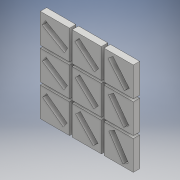
# Autodesk Inventor part: magnet-54-offset-9
Saved by Autodesk Inventor 2018 (Build 220112000, 112)
## iProperties
Created: 2025-03-17
Part Number: magnet-54-offset-9
Material: Generic
Document SubType Name: Modeling
Designer: neo
Density: 1 g/cm^3
Appearance: Default
Author: neo
Autodesk Inventor part; units mm, degrees
ref_plane "YZ Plane" through (0, 0, 0) normal (1, 0, 0) x (0, 1, 0)
ref_plane "XZ Plane" through (0, 0, 0) normal (0, 1, 0) x (-1, 0, 0)
ref_plane "XY Plane" through (0, 0, 0) normal (0, 0, 1) x (1, 0, 0)
sketch "Sketch1" plane through (0, 0, 0) normal (0, 1, 0) x (-1, 0, 0)
  line L0 (44.286, 57.5056) -> (-1.714, 57.5056)
  line L1 (-1.714, 57.5056) -> (-1.714, 11.5056)
  line L2 (-1.714, 11.5056) -> (44.286, 11.5056)
  line L3 (44.286, 11.5056) -> (44.286, 57.5056)
  line L4 (21.286, 57.5056) -> (21.286, 11.5056) construction
  line L5 (44.286, 34.5056) -> (-1.714, 34.5056) construction
  line L6 (32.0821, 50.9202) -> (21.286, 34.5056) construction
  line L7 (21.286, 34.5056) -> (12.8023, 40.0854) construction
  line L8 (36.6614, 48.5107) -> (28.0558, 54.1706)
  line L9 (28.0558, 54.1706) -> (5.9106, 20.5005)
  line L10 (5.9106, 20.5005) -> (14.5162, 14.8405)
  line L11 (14.5162, 14.8405) -> (36.6614, 48.5107)
  line L12 (94.286, 57.5056) -> (48.286, 57.5056)
  line L13 (48.286, 57.5056) -> (48.286, 11.5056)
  line L14 (48.286, 11.5056) -> (94.286, 11.5056)
  line L15 (94.286, 11.5056) -> (94.286, 57.5056)
  line L16 (71.286, 57.5056) -> (71.286, 11.5056) construction
  line L17 (94.286, 34.5056) -> (48.286, 34.5056) construction
  line L18 (84.7685, 48.7961) -> (71.286, 34.5056) construction
  line L19 (71.286, 34.5056) -> (63.9001, 41.4738) construction
  line L20 (88.8597, 45.628) -> (81.3678, 52.6963)
  line L21 (81.3678, 52.6963) -> (53.7123, 23.3831)
  line L22 (53.7123, 23.3831) -> (61.2042, 16.3148)
  line L23 (61.2042, 16.3148) -> (88.8597, 45.628)
  line L24 (144.286, 57.5056) -> (98.286, 57.5056)
  line L25 (98.286, 57.5056) -> (98.286, 11.5056)
  line L26 (98.286, 11.5056) -> (144.286, 11.5056)
  line L27 (144.286, 11.5056) -> (144.286, 57.5056)
  line L28 (121.286, 57.5056) -> (121.286, 11.5056) construction
  line L29 (144.286, 34.5056) -> (98.286, 34.5056) construction
  line L30 (137.0452, 46.2378) -> (121.286, 34.5056) construction
  line L31 (121.286, 34.5056) -> (115.2223, 42.6505) construction
  line L32 (140.5241, 42.4074) -> (134.3734, 50.6693)
  line L33 (134.3734, 50.6693) -> (102.0478, 26.6038)
  line L34 (102.0478, 26.6038) -> (108.1986, 18.3419)
  line L35 (108.1986, 18.3419) -> (140.5241, 42.4074)
  line L36 (44.286, 107.5056) -> (-1.714, 107.5056)
  line L37 (-1.714, 107.5056) -> (-1.714, 61.5056)
  line L38 (-1.714, 61.5056) -> (44.286, 61.5056)
  line L39 (44.286, 61.5056) -> (44.286, 107.5056)
  line L40 (21.286, 107.5056) -> (21.286, 61.5056) construction
  line L41 (44.286, 84.5056) -> (-1.714, 84.5056) construction
  line L42 (33.0183, 100.2647) -> (21.286, 84.5056) construction
  line L43 (21.286, 84.5056) -> (13.141, 90.5693) construction
  line L44 (37.4497, 97.593) -> (29.1878, 103.7437)
  line L45 (29.1878, 103.7437) -> (5.1223, 71.4182)
  line L46 (5.1223, 71.4182) -> (13.3842, 65.2674)
  line L47 (13.3842, 65.2674) -> (37.4497, 97.593)
  line L48 (44.286, 157.5056) -> (-1.714, 157.5056)
  line L49 (-1.714, 157.5056) -> (-1.714, 111.5056)
  line L50 (-1.714, 111.5056) -> (44.286, 111.5056)
  line L51 (44.286, 111.5056) -> (44.286, 157.5056)
  line L52 (21.286, 157.5056) -> (21.286, 111.5056) construction
  line L53 (44.286, 134.5056) -> (-1.714, 134.5056) construction
  line L54 (33.9147, 149.5559) -> (21.286, 134.5056) construction
  line L55 (21.286, 134.5056) -> (13.5074, 141.0326) construction
  line L56 (38.1833, 146.631) -> (30.293, 153.2517)
  line L57 (30.293, 153.2517) -> (4.3887, 122.3801)
  line L58 (4.3887, 122.3801) -> (12.279, 115.7594)
  line L59 (12.279, 115.7594) -> (38.1833, 146.631)
  line L60 (94.286, 107.5056) -> (48.286, 107.5056)
  line L61 (48.286, 107.5056) -> (48.286, 61.5056)
  line L62 (48.286, 61.5056) -> (94.286, 61.5056)
  line L63 (94.286, 61.5056) -> (94.286, 107.5056)
  line L64 (71.286, 107.5056) -> (71.286, 61.5056) construction
  line L65 (94.286, 84.5056) -> (48.286, 84.5056) construction
  line L66 (85.5766, 97.988) -> (71.286, 84.5056) construction
  line L67 (71.286, 84.5056) -> (64.3177, 91.8915) construction
  line L68 (89.4767, 94.5874) -> (82.4084, 102.0793)
  line L69 (82.4084, 102.0793) -> (53.0953, 74.4238)
  line L70 (53.0953, 74.4238) -> (60.1636, 66.9318)
  line L71 (60.1636, 66.9318) -> (89.4767, 94.5874)
  line L72 (94.286, 157.5056) -> (48.286, 157.5056)
  line L73 (48.286, 157.5056) -> (48.286, 111.5056)
  line L74 (48.286, 111.5056) -> (94.286, 111.5056)
  line L75 (94.286, 111.5056) -> (94.286, 157.5056)
  line L76 (71.286, 157.5056) -> (71.286, 111.5056) construction
  line L77 (94.286, 134.5056) -> (48.286, 134.5056) construction
  line L78 (86.3363, 147.1343) -> (71.286, 134.5056) construction
  line L79 (71.286, 134.5056) -> (64.759, 142.2842) construction
  line L80 (90.0321, 143.5126) -> (83.4114, 151.4029)
  line L81 (83.4114, 151.4029) -> (52.5398, 125.4985)
  line L82 (52.5398, 125.4985) -> (59.1606, 117.6083)
  line L83 (59.1606, 117.6083) -> (90.0321, 143.5126)
  line L84 (144.286, 107.5056) -> (98.286, 107.5056)
  line L85 (98.286, 107.5056) -> (98.286, 61.5056)
  line L86 (98.286, 61.5056) -> (144.286, 61.5056)
  line L87 (144.286, 61.5056) -> (144.286, 107.5056)
  line L88 (121.286, 107.5056) -> (121.286, 61.5056) construction
  line L89 (144.286, 84.5056) -> (98.286, 84.5056) construction
  line L90 (137.7007, 95.3017) -> (121.286, 84.5056) construction
  line L91 (121.286, 84.5056) -> (115.7062, 92.9893) construction
  line L92 (140.951, 91.2754) -> (135.2911, 99.8809)
  line L93 (135.2911, 99.8809) -> (101.6209, 77.7357)
  line L94 (101.6209, 77.7357) -> (107.2809, 69.1302)
  line L95 (107.2809, 69.1302) -> (140.951, 91.2754)
  line L96 (144.286, 157.5056) -> (98.286, 157.5056)
  line L97 (98.286, 157.5056) -> (98.286, 111.5056)
  line L98 (98.286, 111.5056) -> (144.286, 111.5056)
  line L99 (144.286, 111.5056) -> (144.286, 157.5056)
  line L100 (121.286, 157.5056) -> (121.286, 111.5056) construction
  line L101 (144.286, 134.5056) -> (98.286, 134.5056) construction
  line L102 (138.3006, 144.329) -> (121.286, 134.5056) construction
  line L103 (121.286, 134.5056) -> (116.2089, 143.2994) construction
  line L104 (141.3114, 140.1205) -> (136.1614, 149.0406)
  line L105 (136.1614, 149.0406) -> (101.2606, 128.8906)
  line L106 (101.2606, 128.8906) -> (106.4106, 119.9705)
  line L107 (106.4106, 119.9705) -> (141.3114, 140.1205)
  dimension "w" = 46
  dimension "d65" = 46
  dimension "d" = 10.3
  dimension "d67" = 40.3
  dimension "d68" = 56.667
  dimension "d69" = 46
  dimension "d70" = 46
  dimension "d71" = 10.3
  dimension "d72" = 40.3
  dimension "d73" = 46.667
  dimension "d76" = 46
  dimension "d77" = 46
  dimension "d78" = 10.3
  dimension "d79" = 40.3
  dimension "d80" = 36.667
  dimension "d83" = 46
  dimension "d84" = 46
  dimension "d85" = 10.3
  dimension "d86" = 40.3
  dimension "d87" = 53.333
  dimension "d90" = 46
  dimension "d91" = 46
  dimension "d92" = 10.3
  dimension "d93" = 40.3
  dimension "d94" = 50
  dimension "d97" = 46
  dimension "d98" = 46
  dimension "d99" = 10.3
  dimension "d100" = 40.3
  dimension "d101" = 43.333
  dimension "d104" = 46
  dimension "d105" = 46
  dimension "d106" = 10.3
  dimension "d107" = 40.3
  dimension "d108" = 40
  dimension "d111" = 46
  dimension "d112" = 46
  dimension "d113" = 10.3
  dimension "d114" = 40.3
  dimension "d115" = 33.333
  dimension "d118" = 46
  dimension "d119" = 46
  dimension "d120" = 10.3
  dimension "d121" = 40.3
  dimension "d122" = 30
  constraints: 216 end point, 45 midpoint, 36 perpendicular, 18 equal length, 18 parallel, 9 horizontal, 18 other
  measures "w" distance of L2.end L0.start
  measures "d65" distance of L0.start L0.end
  measures "d" distance between parallel lines of L9 L11
  measures "d67" distance between parallel lines of L10 L8
  measures "d68" angle of L5 L6
  measures "d69" distance of L14.end L12.start
  measures "d70" distance of L12.start L12.end
  measures "d71" distance between parallel lines of L21 L23
  measures "d72" distance between parallel lines of L22 L20
  measures "d73" angle of L17 L18
  measures "d76" distance of L26.end L24.start
  measures "d77" distance of L24.start L24.end
  measures "d78" distance between parallel lines of L33 L35
  measures "d79" distance between parallel lines of L34 L32
  measures "d80" angle of L29 L30
  measures "d83" distance of L38.end L36.start
  measures "d84" distance of L36.start L36.end
  measures "d85" distance between parallel lines of L45 L47
  measures "d86" distance between parallel lines of L46 L44
  measures "d87" angle of L41 L42
  measures "d90" distance of L50.end L48.start
  measures "d91" distance of L48.start L48.end
  measures "d92" distance between parallel lines of L57 L59
  measures "d93" distance between parallel lines of L58 L56
  measures "d94" angle of L53 L54
  measures "d97" distance of L62.end L60.start
  measures "d98" distance of L60.start L60.end
  measures "d99" distance between parallel lines of L69 L71
  measures "d100" distance between parallel lines of L70 L68
  measures "d101" angle of L65 L66
  measures "d104" distance of L74.end L72.start
  measures "d105" distance of L72.start L72.end
  measures "d106" distance between parallel lines of L81 L83
  measures "d107" distance between parallel lines of L82 L80
  measures "d108" angle of L77 L78
  measures "d111" distance of L86.end L84.start
  measures "d112" distance of L84.start L84.end
  measures "d113" distance between parallel lines of L93 L95
  measures "d114" distance between parallel lines of L94 L92
  measures "d115" angle of L89 L90
  measures "d118" distance of L98.end L96.start
  measures "d119" distance of L96.start L96.end
  measures "d120" distance between parallel lines of L105 L107
  measures "d121" distance between parallel lines of L106 L104
  measures "d122" angle of L101 L102
extrude "Extrusion1" add sketch "Sketch1" along normal blind 10
equation "\"d68\" = a0 + 8 * ad"
equation "\"d73\" = a0 + 5 * ad"
equation "\"d80\" = a0 + 2 * ad"
equation "\"d87\" = a0 + 7 * ad"
equation "\"d94\" = a0 + 6 * ad"
equation "\"d101\" = a0 + 4 * ad"
equation "\"d108\" = a0 + 3 * ad"
equation "\"d115\" = a0 + ad"
equation "\"d122\" = a0 + 0 * ad"
equation "\"ad\" = 3.33333deg"
equation "\"a0\" = 9 * ad"
equation "\"d74\" = 0 * d75"
equation "\"d75\" = 3.333333deg"
equation "\"d81\" = 0 * d82"
equation "\"d82\" = 3.333333deg"
equation "\"d88\" = 0 * d89"
equation "\"d89\" = 3.333333deg"
equation "\"d95\" = 0 * d96"
equation "\"d96\" = 3.333333deg"
equation "\"d102\" = 0 * d103"
equation "\"d103\" = 3.333333deg"
equation "\"d109\" = 0 * d110"
equation "\"d110\" = 3.333333deg"
equation "\"d116\" = 0 * d117"
equation "\"d117\" = 3.333333deg"
equation "\"d123\" = 0 * d124"
equation "\"d124\" = 3.333333deg"
body "Solid1"
